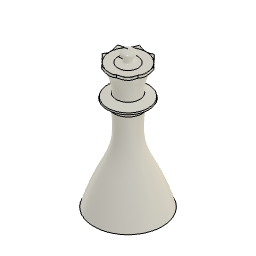
Queen v3 (Autodesk Fusion 360 design; units mm, degrees)
Autodesk Fusion 360 part; units mm, degrees
sketch "Sketch1" plane through (0, 0, 0) normal (0, 1, 0) x (1, 0, 0)
  line L0 (0, 0) -> (0, -85)
  line L1 (0, 0) -> (-21.25, 0)
  spline S0 degree 5 poles (-21.25, 0) (-20.5462, -2.3433) (-19.1499, -6.7502) (-17.0895, -12.5209) (-14.4454, -18.6826) (-11.5056, -24.6083) (-9.1582, -29.6604) (-7.603, -34.6438) (-6.9084, -39.9689) (-6.9734, -45.5239) (-7.2538, -50.0318) (-7.6365, -52.5133) (-8.0931, -53.7597) (-8.4928, -54.335) (-8.7164, -54.5586) knots 0 0 0 0 0 0 0.1 0.2 0.3 0.4 0.5 0.6 0.7 0.8 0.9 1 1 1 1 1 1
  line L2 (-7.02, -37.2676) -> (-6.98, -48.7324)
  line L3 (-24.4738, 10.7337) -> (-18.0262, -10.7337)
  line L4 (-12.8771, -58.7193) -> (-8.7164, -54.5586)
  line L5 (-12.638, -59.5462) -> (-12.8771, -58.7193)
  line L6 (-7.343, -61.5169) -> (-12.638, -59.5462)
  line L7 (-6.8181, -52.6603) -> (-10.6147, -56.4569)
  spline S1 degree 5 poles (-13.1569, -78.5027) (-12.4892, -77.7088) (-11.2807, -76.1544) (-9.8487, -73.923) (-8.5957, -71.1204) (-7.7576, -67.8087) (-7.4445, -65.2532) (-7.3447, -63.3722) (-7.3342, -62.1329) (-7.343, -61.5169) knots 0 0 0 0 0 0 0.2 0.4 0.6 0.8 1 1 1 1 1 1
  line L8 (-14.6843, -80.3185) -> (-11.6296, -76.6868)
  line L9 (-13.1569, -78.5027) -> (-12.3917, -79.1464)
  line L10 (-11.3516, -77.8444) -> (0, -77.8444)
  spline S2 degree 3 poles (-12.3917, -79.1464) (-12.0221, -78.707) (-11.676, -78.2731) (-11.3516, -77.8444) knots 0 0 0 0 0.067818 0.067818 0.067818 0.067818
  spline S3 degree 5 poles (0, -85) (-0.2704, -85) (-0.7932, -84.9807) (-1.5236, -84.8938) (-2.3815, -84.6694) (-3.2166, -84.2487) (-3.7573, -83.7253) (-3.9628, -83.1299) (-3.7936, -82.4359) (-3.3163, -81.6293) (-2.7424, -80.7887) (-2.2901, -79.9992) (-2.1518, -79.3422) (-2.3237, -78.8165) (-2.7541, -78.3928) (-3.493, -78.0775) (-4.3771, -77.9184) (-5.2343, -77.8579) (-5.8959, -77.8444) (-6.2493, -77.8444) knots 0 0 0 0 0 0 0.066667 0.133333 0.2 0.266667 0.333333 0.4 0.466667 0.533333 0.6 0.666667 0.733333 0.8 0.866667 0.933333 1 1 1 1 1 1
  line L11 (-3.9297, -77.8444) -> (-8.5689, -77.8444)
  line L12 (-2.2286, -80.1018) -> (-2.2286, -78.7046)
  line L13 (-3.8706, -83.8443) -> (-3.8706, -82.2964)
  line L14 (1.7404, -85) -> (-1.7404, -85)
  line L15 (-5.25, 0) -> (-5.25, -2.5)
  line L16 (-5.25, -2.5) -> (0, -2.5)
  point P0 (-7, -43)
  point P1 (-3.8706, -83.0703)
  point P2 (-2.2286, -79.4032)
  dimension "d1" = 85
  dimension "d2" = 21.25
  dimension "d3" = 45
  dimension "d14" = 2.5
  dimension "d15" = 5.25
  constraint coincident L0.start L1.start
  constraint vertical L0
  constraint perpendicular L0 L1
  constraint midpoint P0 L2
  constraint midpoint L1.end L3
  constraint midpoint S0.end L7
  constraint parallel L4 L7
  constraint midpoint S1.start L8
  constraint coincident L0 L10.end
  constraint perpendicular L0 L10
  constraint coincident L10 S3.end
  constraint midpoint S3.end L11
  constraint parallel L10 L11
  constraint midpoint P2 L12
  constraint parallel L0 L12
  constraint midpoint P1 L13
  constraint parallel L0 L13
  constraint midpoint L0.end L14
  constraint perpendicular L0 L14
  constraint coincident L1 L15.start
  constraint perpendicular L1 L15
  constraint coincident L0 L16.end
  constraint perpendicular L0 L16
  measures "d1" distance of L0.start L0.end
  measures "d2" distance of L0.start L1.end
  measures "d3" angle of L0 L4
  measures "d14" distance of L15.start L15.end
  measures "d15" distance of L15.end L16.end
revolve "Revolve1" add sketch "Sketch1" angle 360 about axis through (0, 0, 0) along (0, 0, 1) contours L0 L1 S0 L4 L5 L6 L7 S1 L9 L10 S2 L11 L15 L16 | L0 L10 S3 L11
sketch "Sketch3" plane through (0, 0, 0) normal (0, 0, 1) x (1, 0, 0)
  line L0 (0, 0) -> (0, 11.3516) construction
  line L1 (0, 11.3516) -> (0, 13.1569) construction
  circle A0 centre (0, 0) radius 13.1569
  circle A1 centre (0, 0) radius 11.3516 construction
  spline S0 degree 5 poles (-8.242, 10.2554) (-7.917, 10.5166) (-7.2759, 10.9649) (-6.3405, 11.4151) (-5.1187, 11.6257) (-3.4944, 11.5235) (-1.6638, 11.3506) (0.4217, 11.3289) (2.5464, 11.4125) (4.5486, 11.4203) (6.3999, 11.1591) (7.7699, 10.5717) (8.7526, 9.8467) (9.3907, 9.2269) (9.7056, 8.883) knots 0 0 0 0 0 0 0.1 0.2 0.3 0.4 0.5 0.6 0.7 0.8 0.9 1 1 1 1 1 1
  line L2 (9.368, 9.2518) -> (10.0431, 8.5141)
  line L3 (-8.6318, 9.9422) -> (-7.8523, 10.5686)
  line L4 (-0.5, 11.3511) -> (0.5, 11.3521)
  dimension "d9" = 18
  dimension "d12" = 1
  dimension "d13" = 1
  constraint coincident L0.start A0.centre
  constraint vertical L0
  constraint parallel L0 L1
  constraint coincident L1.end A0
  constraint coincident L0.end A1
  constraint coincident A0 S0.start
  constraint coincident A0 S0.end
  constraint midpoint S0.end L2
  constraint tangent A0 L2
  constraint midpoint S0.start L3
  constraint tangent A0 L3
  constraint midpoint L0.end L4
  constraint tangent A1 L4
  constraint equal L2 L3
  measures "d9" distance of S0.start S0.end
  measures "d12" distance of L2.start L2.end
  measures "d13" horizontal distance of L4.start L4.end
extrude "Extrude1" cut sketch "Sketch3" along normal blind 10 from surface at 75 contours A0 S0 picked at (0.7318, 11.832)
pattern_circular "C-Pattern1" count 8 over 360 about axis through (0, 0, 1.75) along (0, 0, 1) of "Extrude1"
equation "d2 = 1 / 4 * d1"
